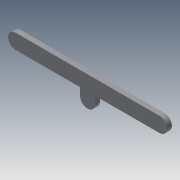
# Autodesk Inventor part: tahlo6_sablona
Saved by Autodesk Inventor 2013 (Build 170138000, 138)
## iProperties
Created: 2013-03-29
Part Number: tahlo6_sablona
Material: Generic
Document SubType Name: Modeling
Designer: idle-rug
Density: 1 g/cm^3
Author: idle-rug
Autodesk Inventor part; units mm, degrees
ref_plane "YZ Plane" through (0, 0, 0) normal (1, 0, 0) x (0, 1, 0)
ref_plane "XZ Plane" through (0, 0, 0) normal (0, 1, 0) x (-1, 0, 0)
ref_plane "XY Plane" through (0, 0, 0) normal (0, 0, 1) x (1, 0, 0)
sketch "Sketch1" plane through (0, 0, 0) normal (0, 1, 0) x (-1, 0, 0)
  line L0 (-9, -3) -> (9, -3)
  line L1 (9, -3) -> (9, 3)
  line L2 (9, 3) -> (-9, 3)
  line L3 (-9, 3) -> (-9, -3)
  line L4 (-9, -3) -> (9, 3) construction
  line L5 (9, -3) -> (-9, 3) construction
  line L6 (17, -3) -> (17, 3)
  line L7 (9, 3) -> (9, -3)
  line L8 (29, -3) -> (29, 3)
  line L9 (17, 3) -> (17, -3)
  line L10 (-17, -3) -> (-17, 3)
  line L11 (-9, 3) -> (-9, -3)
  line L12 (-29, -3) -> (-29, 3)
  line L13 (-17, 3) -> (-17, -3)
  circle A0 centre (29, 0) radius 3
  circle A1 centre (-29, 0) radius 3
  line L14 (9.01, -3) -> (9.01, 3)
  line L15 (9, 3) -> (9, -3)
  line L16 (9.01, -3) -> (17, -3)
  line L17 (9.01, 3) -> (17, 3)
  line L18 (17.01, -3) -> (17.01, 3)
  line L19 (17, 3) -> (17, -3)
  line L20 (17.01, -3) -> (29, -3)
  line L21 (17.01, 3) -> (29, 3)
  line L22 (-9.01, -3) -> (-9.01, 3)
  line L23 (-9, 3) -> (-9, -3)
  line L24 (-9.01, -3) -> (-17, -3)
  line L25 (-9.01, 3) -> (-17, 3)
  line L26 (-17.01, -3) -> (-17.01, 3)
  line L27 (-17, 3) -> (-17, -3)
  line L28 (-17.01, 3) -> (-29, 3)
  line L29 (-17.01, -3) -> (-29, -3)
  line L30 (0, -3) -> (0, -6)
  circle A2 centre (0, -6) radius 3
  line L31 (-3, -6) -> (3, -6)
  line L32 (3, -6) -> (3, -3)
  line L33 (3, -3) -> (-3, -3)
  line L34 (-3, -3) -> (-3, -6)
  line L35 (-3, -6) -> (3, -3) construction
  line L36 (3, -6) -> (-3, -3) construction
  point P0 (0, 0)
  point P1 (0, -4.5)
  dimension "d17" = 18
  dimension "d18" = 6
  dimension "d19" = 8
  dimension "d20" = 12
  dimension "d21" = 8
  dimension "d22" = 12
  dimension "d23" = 0.01
  dimension "d24" = 0.01
  dimension "d25" = 0.01
  dimension "d26" = 0.01
  dimension "d27" = 3
  constraints: 74 end point, 15 parallel, 8 midpoint, 6 horizontal, 6 perpendicular, 3 vertical alignment, 1 coincident, 1 point on line, 6 other
  measures "d17" distance of L2.end L1.end
  measures "d18" distance of L1.end L0.end
  measures "d19" distance of L7.start L6.end
  measures "d20" distance of L9.start L8.end
  measures "d21" distance of L10.end L11.start
  measures "d22" distance of L12.end L13.start
  measures "d23" distance of L15.start L14.end
  measures "d24" distance of L19.start L18.end
  measures "d25" distance of L22.end L23.start
  measures "d26" distance of L26.end L27.start
  measures "d27" distance of L30.start L30.end
extrude "Extrusion1" add sketch "Sketch1" along normal blind 2
sketch "Sketch2" plane through (0, 2, 0) normal (0, 1, 0) x (1, 0, 0)
  arc A0 (3, 6) -> (-3, 6) centre (0, 6) ccw projected
  circle A1 centre (0, 6) radius 0.05
  circle A2 centre (0, 0) radius 0.05
  dimension "d30" = 0.1
  dimension "d31" = 0.1
  constraints: 2 centre point, 2 coincident
  measures "d30" diameter of A1
  measures "d31" diameter of A2
extrude "Extrusion2" cut sketch "Sketch2" against normal blind 2
sketch "Sketch3" plane through (0, 2, 0) normal (0, 1, 0) x (1, 0, 0)
  arc A0 (-29, 3) -> (-29, -3) centre (-29, 0) ccw projected
  circle A1 centre (-29, 0) radius 0.05
  point P0 (0, 0)
  dimension "d34" = 0.1
  constraints: 1 centre point, 1 coincident
  measures "d34" diameter of A1
extrude "Extrusion3" cut sketch "Sketch3" against normal blind 2
sketch "Sketch4" plane through (0, 2, 0) normal (0, 1, 0) x (1, 0, 0)
  arc A0 (29, -3) -> (29, 3) centre (29, 0) ccw projected
  circle A1 centre (29, 0) radius 0.05
  point P0 (0, 0)
  dimension "d37" = 0.1
  constraints: 1 centre point, 1 coincident
  measures "d37" diameter of A1
extrude "Extrusion4" cut sketch "Sketch4" against normal blind 2
body "Solid1"
